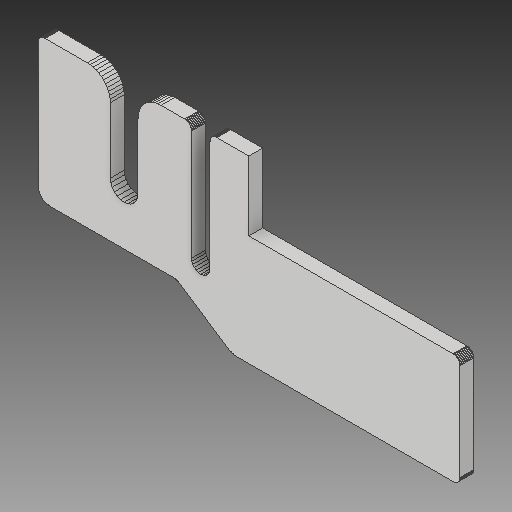
# Autodesk Inventor part: handyDandy
Saved by Autodesk Inventor 2018 (Build 220112000, 112)
## iProperties
Created: 2016-08-18
Part Number: handyDandy
Material: Generic
Document SubType Name: Modeling
Designer: User
Density: 1 g/cm^3
Appearance: Default
Author: User
Autodesk Inventor part; units mm, degrees
ref_plane "YZ Plane" through (0, 0, 0) normal (1, 0, 0) x (0, 1, 0)
ref_plane "XZ Plane" through (0, 0, 0) normal (0, 1, 0) x (-1, 0, 0)
ref_plane "XY Plane" through (0, 0, 0) normal (0, 0, 1) x (1, 0, 0)
sketch "Sketch1" plane through (0, 0, 0) normal (0, 0, 1) x (1, 0, 0)
  line L0 (195.6833, 213.3467) -> (195.5833, 213.7217)
  line L1 (195.5833, 213.7217) -> (195.4583, 214.0967)
  line L2 (195.4583, 214.0967) -> (195.2833, 214.4467)
  line L3 (195.2833, 214.4467) -> (195.0833, 214.7717)
  line L4 (195.0833, 214.7717) -> (194.8083, 215.0717)
  line L5 (194.8083, 215.0717) -> (194.5333, 215.3217)
  line L6 (194.5333, 215.3217) -> (194.2083, 215.5467)
  line L7 (194.2083, 215.5467) -> (193.8333, 215.7217)
  line L8 (193.8333, 215.7217) -> (193.4833, 215.8467)
  line L9 (193.4833, 215.8467) -> (193.0833, 215.9217)
  line L10 (193.0833, 215.9217) -> (192.7083, 215.9467)
  line L11 (192.7083, 215.9467) -> (104.1084, 215.9467)
  line L12 (104.1084, 215.9467) -> (104.1084, 245.9467)
  line L13 (104.1084, 245.9467) -> (90.2583, 245.9467)
  line L14 (90.2583, 245.9467) -> (89.8584, 245.9217)
  line L15 (89.8584, 245.9217) -> (89.4333, 245.8467)
  line L16 (89.4333, 245.8467) -> (89.0333, 245.6967)
  line L17 (89.0333, 245.6967) -> (88.6583, 245.4967)
  line L18 (88.6583, 245.4967) -> (88.3083, 245.2467)
  line L19 (88.3083, 245.2467) -> (88.0083, 244.9467)
  line L20 (88.0083, 244.9467) -> (87.7583, 244.5967)
  line L21 (87.7583, 244.5967) -> (87.5584, 244.2467)
  line L22 (87.5584, 244.2467) -> (87.3833, 243.8467)
  line L23 (87.3833, 243.8467) -> (87.2583, 242.9967)
  line L24 (87.2583, 242.9967) -> (87.2583, 242.5967)
  line L25 (87.2583, 242.5967) -> (87.2583, 195.1217)
  line L26 (87.2583, 195.1217) -> (87.1333, 194.0967)
  line L27 (87.1333, 194.0967) -> (86.7333, 193.1217)
  line L28 (86.7333, 193.1217) -> (86.1083, 192.2967)
  line L29 (86.1083, 192.2967) -> (85.2583, 191.6717)
  line L30 (85.2583, 191.6717) -> (84.3084, 191.2717)
  line L31 (84.3084, 191.2717) -> (83.2583, 191.1217)
  line L32 (83.2583, 191.1217) -> (82.2334, 191.2717)
  line L33 (82.2334, 191.2717) -> (81.2583, 191.6717)
  line L34 (81.2583, 191.6717) -> (80.4333, 192.2967)
  line L35 (80.4333, 192.2967) -> (79.8083, 193.1217)
  line L36 (79.8083, 193.1217) -> (79.4083, 194.0967)
  line L37 (79.4083, 194.0967) -> (79.2583, 195.1217)
  line L38 (79.2583, 195.1217) -> (79.2583, 242.9467)
  line L39 (79.2583, 242.9467) -> (79.2333, 243.3467)
  line L40 (79.2333, 243.3467) -> (79.1583, 243.7217)
  line L41 (79.1583, 243.7217) -> (79.0333, 244.0967)
  line L42 (79.0333, 244.0967) -> (78.8584, 244.4467)
  line L43 (78.8584, 244.4467) -> (78.6583, 244.7717)
  line L44 (78.6583, 244.7717) -> (78.3834, 245.0717)
  line L45 (78.3834, 245.0717) -> (78.1083, 245.3217)
  line L46 (78.1083, 245.3217) -> (77.7583, 245.5467)
  line L47 (77.7583, 245.5467) -> (77.4083, 245.7217)
  line L48 (77.4083, 245.7217) -> (77.0583, 245.8467)
  line L49 (77.0583, 245.8467) -> (76.6583, 245.9217)
  line L50 (76.6583, 245.9217) -> (76.2584, 245.9467)
  line L51 (76.2584, 245.9467) -> (66.0084, 245.9467)
  line L52 (66.0084, 245.9467) -> (64.7083, 245.8717)
  line L53 (64.7083, 245.8717) -> (63.4333, 245.6217)
  line L54 (63.4333, 245.6217) -> (62.1833, 245.1967)
  line L55 (62.1833, 245.1967) -> (61.0083, 244.6217)
  line L56 (61.0083, 244.6217) -> (59.9333, 243.8967)
  line L57 (59.9333, 243.8967) -> (58.9333, 243.0217)
  line L58 (58.9333, 243.0217) -> (58.0833, 242.0467)
  line L59 (58.0833, 242.0467) -> (57.3583, 240.9467)
  line L60 (57.3583, 240.9467) -> (56.7834, 239.7717)
  line L61 (56.7834, 239.7717) -> (56.3583, 238.5467)
  line L62 (56.3583, 238.5467) -> (56.1084, 237.2467)
  line L63 (56.1084, 237.2467) -> (56.0083, 235.9467)
  line L64 (56.0083, 235.9467) -> (56.0083, 207.5467)
  line L65 (56.0083, 207.5467) -> (55.8084, 205.9967)
  line L66 (55.8084, 205.9967) -> (55.2083, 204.5467)
  line L67 (55.2083, 204.5467) -> (54.2584, 203.2967)
  line L68 (54.2584, 203.2967) -> (53.0083, 202.3467)
  line L69 (53.0083, 202.3467) -> (51.5583, 201.7467)
  line L70 (51.5583, 201.7467) -> (50.0083, 201.5467)
  line L71 (50.0083, 201.5467) -> (48.4583, 201.7467)
  line L72 (48.4583, 201.7467) -> (47.0083, 202.3467)
  line L73 (47.0083, 202.3467) -> (45.7583, 203.2967)
  line L74 (45.7583, 203.2967) -> (44.8084, 204.5467)
  line L75 (44.8084, 204.5467) -> (44.2083, 205.9967)
  line L76 (44.2083, 205.9967) -> (44.0084, 207.5467)
  line L77 (44.0084, 207.5467) -> (44.0084, 235.9467)
  line L78 (44.0084, 235.9467) -> (43.9334, 237.2467)
  line L79 (43.9334, 237.2467) -> (43.6833, 238.5467)
  line L80 (43.6833, 238.5467) -> (43.2583, 239.7717)
  line L81 (43.2583, 239.7717) -> (42.6833, 240.9467)
  line L82 (42.6833, 240.9467) -> (41.9583, 242.0467)
  line L83 (41.9583, 242.0467) -> (41.0833, 243.0217)
  line L84 (41.0833, 243.0217) -> (40.1083, 243.8967)
  line L85 (40.1083, 243.8967) -> (39.0083, 244.6217)
  line L86 (39.0083, 244.6217) -> (37.8333, 245.1967)
  line L87 (37.8333, 245.1967) -> (36.6083, 245.6217)
  line L88 (36.6083, 245.6217) -> (35.3083, 245.8717)
  line L89 (35.3083, 245.8717) -> (34.0083, 245.9467)
  line L90 (34.0083, 245.9467) -> (15.7333, 245.9467)
  line L91 (15.7333, 245.9467) -> (15.3333, 245.9217)
  line L92 (15.3333, 245.9217) -> (14.9333, 245.8467)
  line L93 (14.9333, 245.8467) -> (14.5833, 245.7217)
  line L94 (14.5833, 245.7217) -> (14.2333, 245.5467)
  line L95 (14.2333, 245.5467) -> (13.8833, 245.3217)
  line L96 (13.8833, 245.3217) -> (13.6083, 245.0717)
  line L97 (13.6083, 245.0717) -> (13.3333, 244.7717)
  line L98 (13.3333, 244.7717) -> (13.1333, 244.4467)
  line L99 (13.1333, 244.4467) -> (12.9583, 244.0967)
  line L100 (12.9583, 244.0967) -> (12.8333, 243.7217)
  line L101 (12.8333, 243.7217) -> (12.7584, 243.3467)
  line L102 (12.7584, 243.3467) -> (12.7333, 242.9467)
  line L103 (12.7333, 242.9467) -> (12.7333, 188.9467)
  line L104 (12.7333, 188.9467) -> (12.7584, 188.2967)
  line L105 (12.7584, 188.2967) -> (12.8833, 187.6467)
  line L106 (12.8833, 187.6467) -> (13.1083, 187.0467)
  line L107 (13.1083, 187.0467) -> (13.3833, 186.4467)
  line L108 (13.3833, 186.4467) -> (13.7583, 185.8967)
  line L109 (13.7583, 185.8967) -> (14.1833, 185.4217)
  line L110 (14.1833, 185.4217) -> (14.6833, 184.9967)
  line L111 (14.6833, 184.9967) -> (15.2333, 184.6217)
  line L112 (15.2333, 184.6217) -> (15.8083, 184.3217)
  line L113 (15.8083, 184.3217) -> (16.4333, 184.1217)
  line L114 (16.4333, 184.1217) -> (17.0583, 183.9967)
  line L115 (17.0583, 183.9967) -> (17.7333, 183.9467)
  line L116 (17.7333, 183.9467) -> (70.9334, 183.9467)
  line L117 (70.9334, 183.9467) -> (72.0833, 183.8467)
  line L118 (72.0833, 183.8467) -> (72.3584, 183.7717)
  line L119 (72.3584, 183.7717) -> (72.6333, 183.6967)
  line L120 (72.6333, 183.6967) -> (72.9333, 183.5967)
  line L121 (72.9333, 183.5967) -> (73.1833, 183.4967)
  line L122 (73.1833, 183.4967) -> (73.4583, 183.3967)
  line L123 (73.4583, 183.3967) -> (73.7333, 183.2467)
  line L124 (73.7333, 183.2467) -> (74.2333, 182.9717)
  line L125 (74.2333, 182.9717) -> (95.4083, 168.9467)
  line L126 (95.4083, 168.9467) -> (95.9333, 168.6717)
  line L127 (95.9333, 168.6717) -> (96.1833, 168.5467)
  line L128 (96.1833, 168.5467) -> (96.4583, 168.4467)
  line L129 (96.4583, 168.4467) -> (96.7333, 168.3467)
  line L130 (96.7333, 168.3467) -> (97.0084, 168.2467)
  line L131 (97.0084, 168.2467) -> (97.2833, 168.1717)
  line L132 (97.2833, 168.1717) -> (97.5583, 168.1217)
  line L133 (97.5583, 168.1217) -> (97.8583, 168.0467)
  line L134 (97.8583, 168.0467) -> (98.1333, 168.0217)
  line L135 (98.1333, 168.0217) -> (98.7084, 167.9467)
  line L136 (98.7084, 167.9467) -> (192.7083, 167.9467)
  line L137 (192.7083, 167.9467) -> (193.0833, 167.9717)
  line L138 (193.0833, 167.9717) -> (193.4833, 168.0467)
  line L139 (193.4833, 168.0467) -> (193.8333, 168.1717)
  line L140 (193.8333, 168.1717) -> (194.2083, 168.3467)
  line L141 (194.2083, 168.3467) -> (194.5333, 168.5717)
  line L142 (194.5333, 168.5717) -> (194.8083, 168.8217)
  line L143 (194.8083, 168.8217) -> (195.0833, 169.1217)
  line L144 (195.0833, 169.1217) -> (195.2833, 169.4467)
  line L145 (195.2833, 169.4467) -> (195.4583, 169.7967)
  line L146 (195.4583, 169.7967) -> (195.5833, 170.1717)
  line L147 (195.5833, 170.1717) -> (195.6833, 170.5717)
  line L148 (195.6833, 170.5717) -> (195.7083, 170.9467)
  line L149 (195.7083, 170.9467) -> (195.7083, 212.9467)
  line L150 (195.7083, 212.9467) -> (195.6833, 213.3467)
  point P0 (0, 0)
  constraints: 302 end point
extrude "Extrusion1" add sketch "Sketch1" along normal blind 6
body "Solid1"
